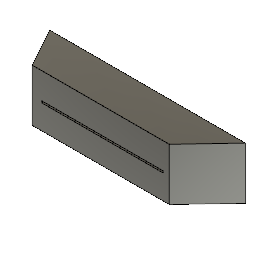
hopper v2 (Autodesk Fusion 360 design; units mm, degrees)
Autodesk Fusion 360 part; units mm, degrees
sketch "hopper" plane through (0, 0, 0) normal (0, 0, 1) x (1, 0, 0)
  line L0 (0, 0) -> (254, 0)
  line L1 (0, 0) -> (-8.4458, 0)
  line L2 (-8.4458, 0) -> (-50, 75)
  line L3 (-50, 75) -> (325, 75)
  line L4 (325, 75) -> (254, 0)
  dimension "d4" = 375
  dimension "d5" = 61.011
  dimension "d6" = 46.569
  dimension "d7" = 75
  dimension "d19" = 262.4458
  constraint coincident L0.start L1.start
  constraint horizontal L3
  measures "d4" distance of L2.end L3.end
  measures "d5" angle of L2 L3
  measures "d6" angle of L3 L4
  measures "d7" vertical distance of L0.end L3.end
  measures "d19" distance of L0.end L1.end
extrude "Extrude1" add sketch "hopper" along normal blind 100
shell "Shell1" thickness 10 removed faces 1 at (75, 75, 33.3333)
sketch "tube slot" plane through (0, 0, 0) normal (0, 1, 0) x (1, 0, 0)
  line L0 (10, -50) -> (241.775, -50)
  line L1 (241.775, -50) -> (241.775, -46.75)
  line L2 (241.775, -46.75) -> (10, -46.75)
  line L3 (10, -46.75) -> (10, -50)
  line L4 (-8.4458, -100) -> (254, -100)
  line L5 (254, 0) -> (254, -100)
  dimension "d11" = 231.775
  dimension "d12" = 3.25
  dimension "d15" = 50
  dimension "d16" = 12.225
  constraint horizontal L0
  constraint vertical L1
  constraint horizontal L2
  constraint vertical L3
  measures "d11" distance of L0.start L0.end
  measures "d12" distance of L0.start L2.end
  measures "d15" distance of L0 L4
  measures "d16" distance of L1.end L5
extrude "Extrude2" cut sketch "tube slot" along normal blind 30
named bodies: "hopper"
